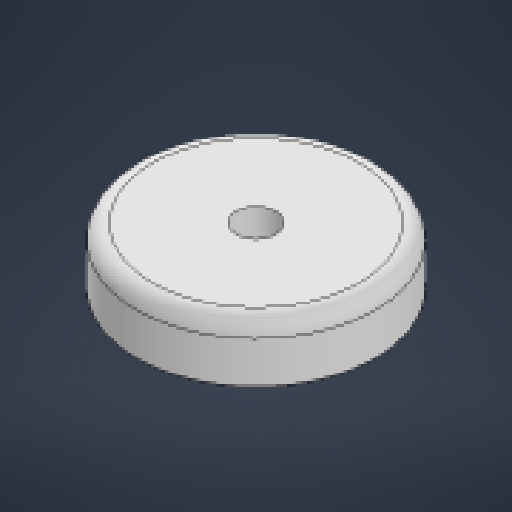
# Autodesk Inventor part: SMALL-MAGNET
Saved by Autodesk Inventor 2026.1 (Build 301233020, 233B)
## iProperties
Created: 2026-03-20
Part Number: SMALL-MAGNET
Material: Steel, Alloy
Document SubType Name: Modeling
Designer: Owen L
Mass: 153.862 g
Surface Area: 53.1858 cm^2
Volume: 19.9045 cm^3
Density: 7.73 g/cm^3
Appearance: Semi-Polished
Author: Owen L
Autodesk Inventor part; units mm, degrees
ref_plane "YZ Plane" through (0, 0, 0) normal (1, 0, 0) x (0, 1, 0)
ref_plane "XZ Plane" through (0, 0, 0) normal (0, 1, 0) x (-1, 0, 0)
ref_plane "XY Plane" through (0, 0, 0) normal (0, 0, 1) x (1, 0, 0)
sketch "Sketch1" plane through (0, 0, 0) normal (0, 0, 1) x (1, 0, 0)
  line L0 (0, 0) -> (0, 7.5879)
  line L1 (-24.0284, 0) -> (-24.0284, 11.557)
  line L2 (-24.0284, 11.557) -> (-4, 11.557)
  line L3 (-4, 11.557) -> (-4, 0)
  line L4 (-24.0284, 0) -> (-4, 0)
  dimension "d0" = 48.0568
  dimension "d2" = 8
  dimension "d3" = 11.557
  constraints: 10 end point, 2 vertical, 1 horizontal, 1 horizontal alignment, 1 perpendicular
  measures "d0" diameter of L1.start L0
  measures "d2" diameter of L3 L0
  measures "d3" distance of L1.start L1.end
revolve "Revolution1" add sketch "Sketch1" angle 360 about axis through (0, 0, 0) along (0, 1, 0)
fillet "Fillet1" radius 3.175 1 edges at (24.0284, 11.557, 0)
chamfer "Chamfer1" distance 3.175 angle 45 1 edges at (4, 0, 0)
body "Solid1"
